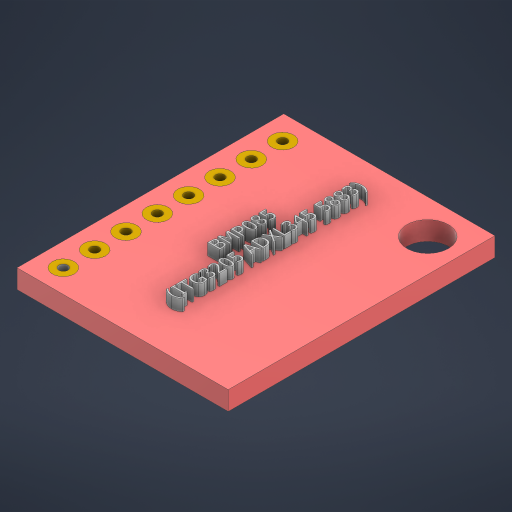
# Autodesk Inventor part: IMU Module
Saved by Autodesk Inventor 2023 (Build 270158000, 158)
## iProperties
Created: 2023-10-20
Part Number: IMU Module
Material: Generic
Document SubType Name: Modeling
Designer: nick_
Density: 1 g/cm^3
Appearance: Default
Author: nick_
Autodesk Inventor part; units mm, degrees
ref_plane "YZ Plane" through (0, 0, 0) normal (1, 0, 0) x (0, 1, 0)
ref_plane "XZ Plane" through (0, 0, 0) normal (0, 1, 0) x (-1, 0, 0)
ref_plane "XY Plane" through (0, 0, 0) normal (0, 0, 1) x (1, 0, 0)
sketch "Sketch1" plane through (0, 0, 0) normal (0, 1, 0) x (-1, 0, 0)
  line L0 (-8.56, 10.81) -> (8.56, 10.81)
  line L1 (8.56, 10.81) -> (8.56, -10.81)
  line L2 (8.56, -10.81) -> (-8.56, -10.81)
  line L3 (-8.56, -10.81) -> (-8.56, 10.81)
  line L4 (-8.56, 10.81) -> (8.56, -10.81) construction
  line L5 (8.56, 10.81) -> (-8.56, -10.81) construction
  point P0 (0, 0)
  dimension "d0" = 17.12
  dimension "d1" = 21.62
  constraints: 12 end point, 2 midpoint, 2 parallel, 1 horizontal, 1 perpendicular
  measures "d0" distance of L1.end L2.end
  measures "d1" distance of L0.end L1.end
extrude "Extrusion1" add sketch "Sketch1" along normal blind 1.53
sketch "Sketch2" plane through (0, 1.53, 0) normal (0, 1, 0) x (1, 0, 0)
  line L0 (8.56, -10.81) -> (8.56, 10.81) projected
  line L1 (8.56, 10.81) -> (-8.56, 10.81) projected
  point P0 (0, 0)
  point P1 (5.895, 8.025)
  dimension "d4" = 2.665
  dimension "d5" = 2.785
  measures "d4" distance from line of L0 point (5.895, 8.025)
  measures "d5" distance from line of L1 point (5.895, 8.025)
hole "Hole1" at (5.895, 1.53, -8.025) direction (0, -1, 0) diameter 3.37 end through all
sketch "Sketch3" plane through (0, 1.53, 0) normal (0, 1, 0) x (1, 0, 0)
  line L0 (-8.56, -10.81) -> (8.56, -10.81) projected
  line L1 (-8.56, 10.81) -> (-8.56, -10.81) projected
  point P0 (0, 0)
  point P1 (-6.685, -8.935)
  dimension "d13" = 1.875
  dimension "d14" = 1.875
  measures "d13" distance from line of L0 point (-6.685, -8.935)
  measures "d14" distance from line of L1 point (-6.685, -8.935)
hole "Hole2" at (-6.685, 1.53, 8.935) direction (0, -1, 0) diameter 0.73 end through all
sketch "Sketch5" plane through (0, 1.53, 0) normal (0, 1, 0) x (1, 0, 0)
  circle A0 centre (-6.685, -8.935) radius 0.365 projected
  circle A1 centre (5.895, 8.025) radius 1.685 construction
  line L0 (8.56, 10.81) -> (-8.56, 10.81) construction
  line L1 (-8.56, 10.81) -> (-8.56, -10.81) construction
  line L2 (-8.56, -10.81) -> (8.56, -10.81) construction
  line L3 (8.56, -10.81) -> (8.56, 10.81) construction
  circle A2 centre (-6.685, -8.935) radius 0.365 construction
  circle A3 centre (-6.685, -8.935) radius 0.885
  point P0 (0, 0)
  dimension "d22" = 1.77
  constraints: 2 coincident, 1 centre point
  measures "d22" diameter of A3
extrude "Extrusion2" add sketch "Sketch5" along normal blind 0.001
pattern_linear "Rectangular Pattern1" count 8 spacing 2.54 along (0, 0, -1) of "Extrusion2", "Hole2"
sketch "Sketch6" plane through (0, 1.53, 0) normal (0, 1, 0) x (1, 0, 0)
  line L0 (-1.7084, -23.5263) -> (-1.7084, 24.1475) construction
  line L1 (-1.7084, 24.1475) -> (7.2695, 24.1475) construction
  line L2 (7.2695, 24.1475) -> (7.2695, -23.5263) construction
  line L3 (7.2695, -23.5263) -> (-1.7084, -23.5263) construction
  spline S0 degree 2 poles (-0.9929, -1.5646) (-0.9183, -1.5646) (-0.804, -1.6213) (-0.7668, -1.6683) knots 0 0 0 1 2 2 2
  spline S1 degree 2 poles (-0.7668, -1.6683) (-0.723, -1.725) (-0.6857, -1.8539) (-0.6857, -1.956) knots 0 0 0 1 2 2 2
  line L4 (-0.6857, -1.956) -> (-0.6857, -2.2429)
  line L5 (-0.6857, -2.2429) -> (-1.6857, -2.2429)
  line L6 (-1.6857, -2.2429) -> (-1.6857, -1.9779)
  spline S2 degree 2 poles (-1.6857, -1.9779) (-1.6857, -1.8709) (-1.672, -1.7639) (-1.6452, -1.7153) knots 0 0 0 1 2 2 2
  spline S3 degree 2 poles (-1.6452, -1.7153) (-1.6169, -1.661) (-1.5237, -1.6116) (-1.4605, -1.6116) knots 0 0 0 1 2 2 2
  spline S4 degree 2 poles (-1.4605, -1.6116) (-1.3899, -1.6116) (-1.2781, -1.6861) (-1.2465, -1.7518) knots 0 0 0 1 2 2 2
  line L7 (-1.2465, -1.7518) -> (-1.2417, -1.7518)
  spline S5 degree 2 poles (-1.2417, -1.7518) (-1.2173, -1.6626) (-1.0885, -1.5646) (-0.9929, -1.5646) knots 0 0 0 1 2 2 2
  spline S6 degree 2 poles (-0.9872, -1.7032) (-1.0439, -1.7032) (-1.1169, -1.7356) (-1.1428, -1.7842) knots 0 0 0 1 2 2 2
  spline S7 degree 2 poles (-1.1428, -1.7842) (-1.159, -1.8158) (-1.1687, -1.8903) (-1.1687, -1.9592) knots 0 0 0 1 2 2 2
  line L8 (-1.1687, -1.9592) -> (-1.1687, -2.11)
  line L9 (-1.1687, -2.11) -> (-0.7992, -2.11)
  line L10 (-0.7992, -2.11) -> (-0.7992, -2.0022)
  spline S8 degree 2 poles (-0.7992, -2.0022) (-0.7992, -1.9147) (-0.8154, -1.8142) (-0.8413, -1.7753) knots 0 0 0 1 2 2 2
  spline S9 degree 2 poles (-0.8413, -1.7753) (-0.8681, -1.738) (-0.9345, -1.7032) (-0.9872, -1.7032) knots 0 0 0 1 2 2 2
  spline S10 degree 2 poles (-1.4418, -1.7502) (-1.4775, -1.7502) (-1.531, -1.7745) (-1.5464, -1.8012) knots 0 0 0 1 2 2 2
  spline S11 degree 2 poles (-1.5464, -1.8012) (-1.5642, -1.8336) (-1.5723, -1.9122) (-1.5723, -1.9827) knots 0 0 0 1 2 2 2
  line L11 (-1.5723, -1.9827) -> (-1.5723, -2.11)
  line L12 (-1.5723, -2.11) -> (-1.2797, -2.11)
  line L13 (-1.2797, -2.11) -> (-1.2797, -1.9592)
  spline S12 degree 2 poles (-1.2797, -1.9592) (-1.2797, -1.8968) (-1.2927, -1.8377) (-1.313, -1.8061) knots 0 0 0 1 2 2 2
  spline S13 degree 2 poles (-1.313, -1.8061) (-1.3324, -1.7753) (-1.3948, -1.7502) (-1.4418, -1.7502) knots 0 0 0 1 2 2 2
  line L14 (-0.6857, -0.5751) -> (-0.6857, -0.708)
  line L15 (-0.6857, -0.708) -> (-1.5472, -0.708)
  line L16 (-1.5472, -0.708) -> (-0.9613, -0.969)
  line L17 (-0.9613, -0.969) -> (-0.9613, -1.05)
  line L18 (-0.9613, -1.05) -> (-1.5472, -1.3085)
  line L19 (-1.5472, -1.3085) -> (-0.6857, -1.3085)
  line L20 (-0.6857, -1.3085) -> (-0.6857, -1.4325)
  line L21 (-0.6857, -1.4325) -> (-1.6857, -1.4325)
  line L22 (-1.6857, -1.4325) -> (-1.6857, -1.251)
  line L23 (-1.6857, -1.251) -> (-1.129, -1.0014)
  line L24 (-1.129, -1.0014) -> (-1.6857, -0.7599)
  line L25 (-1.6857, -0.7599) -> (-1.6857, -0.5751)
  line L26 (-1.6857, -0.5751) -> (-0.6857, -0.5751)
  spline S14 degree 2 poles (-1.3843, 0.2596) (-1.3194, 0.2596) (-1.2028, 0.2134) (-1.1622, 0.172) knots 0 0 0 1 2 2 2
  spline S15 degree 2 poles (-1.1622, 0.172) (-1.1112, 0.1202) (-1.0585, -0.02) (-1.0585, -0.127) knots 0 0 0 1 2 2 2
  line L27 (-1.0585, -0.127) -> (-1.0585, -0.2396)
  line L28 (-1.0585, -0.2396) -> (-0.6857, -0.2396)
  line L29 (-0.6857, -0.2396) -> (-0.6857, -0.3725)
  line L30 (-0.6857, -0.3725) -> (-1.6857, -0.3725)
  line L31 (-1.6857, -0.3725) -> (-1.6857, -0.1213)
  spline S16 degree 2 poles (-1.6857, -0.1213) (-1.6857, -0.0322) (-1.6566, 0.0926) (-1.6233, 0.1404) knots 0 0 0 1 2 2 2
  spline S17 degree 2 poles (-1.6233, 0.1404) (-1.5852, 0.1964) (-1.4677, 0.2596) (-1.3843, 0.2596) knots 0 0 0 1 2 2 2
  spline S18 degree 2 poles (-1.3802, 0.121) (-1.4321, 0.121) (-1.5083, 0.0853) (-1.5326, 0.0489) knots 0 0 0 1 2 2 2
  spline S19 degree 2 poles (-1.5326, 0.0489) (-1.5536, 0.0173) (-1.5707, -0.067) (-1.5707, -0.1294) knots 0 0 0 1 2 2 2
  line L32 (-1.5707, -0.1294) -> (-1.5707, -0.2396)
  line L33 (-1.5707, -0.2396) -> (-1.172, -0.2396)
  line L34 (-1.172, -0.2396) -> (-1.172, -0.1489)
  spline S20 degree 2 poles (-1.172, -0.1489) (-1.172, -0.0678) (-1.1979, 0.0319) (-1.2319, 0.0643) knots 0 0 0 1 2 2 2
  spline S21 degree 2 poles (-1.2319, 0.0643) (-1.2619, 0.0943) (-1.3324, 0.121) (-1.3802, 0.121) knots 0 0 0 1 2 2 2
  spline S22 degree 2 poles (-1.1857, 0.98) (-0.9167, 0.98) (-0.6647, 0.8236) (-0.6647, 0.6607) knots 0 0 0 1 2 2 2
  spline S23 degree 2 poles (-0.6647, 0.6607) (-0.6647, 0.4954) (-0.9216, 0.3406) (-1.1849, 0.3406) knots 0 0 0 1 2 2 2
  spline S24 degree 2 poles (-1.1849, 0.3406) (-1.4556, 0.3406) (-1.706, 0.497) (-1.706, 0.6607) knots 0 0 0 1 2 2 2
  spline S25 degree 2 poles (-1.706, 0.6607) (-1.706, 0.8252) (-1.4467, 0.98) (-1.1857, 0.98) knots 0 0 0 1 2 2 2
  spline S26 degree 2 poles (-0.881, 0.8082) (-0.9305, 0.8276) (-1.0828, 0.8438) (-1.1857, 0.8438) knots 0 0 0 1 2 2 2
  spline S27 degree 2 poles (-1.1857, 0.8438) (-1.2887, 0.8438) (-1.4402, 0.8276) (-1.4912, 0.8074) knots 0 0 0 1 2 2 2
  spline S28 degree 2 poles (-1.4912, 0.8074) (-1.5423, 0.7871) (-1.595, 0.7166) (-1.595, 0.6607) knots 0 0 0 1 2 2 2
  spline S29 degree 2 poles (-1.595, 0.6607) (-1.595, 0.6048) (-1.5423, 0.5327) (-1.4896, 0.5116) knots 0 0 0 1 2 2 2
  spline S30 degree 2 poles (-1.4896, 0.5116) (-1.4386, 0.4913) (-1.283, 0.4767) (-1.1849, 0.4767) knots 0 0 0 1 2 2 2
  spline S31 degree 2 poles (-1.1849, 0.4767) (-1.0796, 0.4767) (-0.9386, 0.4897) (-0.8835, 0.5108) knots 0 0 0 1 2 2 2
  spline S32 degree 2 poles (-0.8835, 0.5108) (-0.8316, 0.5302) (-0.7757, 0.6024) (-0.7757, 0.6607) knots 0 0 0 1 2 2 2
  spline S33 degree 2 poles (-0.7757, 0.6607) (-0.7757, 0.7158) (-0.8284, 0.7879) (-0.881, 0.8082) knots 0 0 0 1 2 2 2
  spline S34 degree 2 poles (-0.663, 1.4103) (-0.663, 1.3357) (-0.7076, 1.2134) (-0.7489, 1.1704) knots 0 0 0 1 2 2 2
  spline S35 degree 2 poles (-0.7489, 1.1704) (-0.7895, 1.1283) (-0.8997, 1.0845) (-0.9621, 1.0845) knots 0 0 0 1 2 2 2
  spline S36 degree 2 poles (-0.9621, 1.0845) (-1.0431, 1.0845) (-1.1793, 1.1712) (-1.2198, 1.2539) knots 0 0 0 1 2 2 2
  line L35 (-1.2198, 1.2539) -> (-1.2238, 1.2539)
  spline S37 degree 2 poles (-1.2238, 1.2539) (-1.2668, 1.1802) (-1.3689, 1.1088) (-1.4451, 1.1088) knots 0 0 0 1 2 2 2
  spline S38 degree 2 poles (-1.4451, 1.1088) (-1.5577, 1.1088) (-1.7084, 1.279) (-1.7084, 1.4103) knots 0 0 0 1 2 2 2
  spline S39 degree 2 poles (-1.7084, 1.4103) (-1.7084, 1.5464) (-1.5658, 1.7109) (-1.454, 1.7109) knots 0 0 0 1 2 2 2
  spline S40 degree 2 poles (-1.454, 1.7109) (-1.3867, 1.7109) (-1.2554, 1.6323) (-1.2181, 1.5586) knots 0 0 0 1 2 2 2
  line L36 (-1.2181, 1.5586) -> (-1.2141, 1.5586)
  spline S41 degree 2 poles (-1.2141, 1.5586) (-1.1736, 1.6461) (-1.0569, 1.7361) (-0.9645, 1.7361) knots 0 0 0 1 2 2 2
  spline S42 degree 2 poles (-0.9645, 1.7361) (-0.8365, 1.7361) (-0.663, 1.5497) (-0.663, 1.4103) knots 0 0 0 1 2 2 2
  spline S43 degree 2 poles (-0.9515, 1.5983) (-1.0131, 1.5983) (-1.0861, 1.5497) (-1.1233, 1.4808) knots 0 0 0 1 2 2 2
  spline S44 degree 2 poles (-1.1233, 1.4808) (-1.1363, 1.4581) (-1.1663, 1.3819) (-1.1857, 1.3341) knots 0 0 0 1 2 2 2
  spline S45 degree 2 poles (-1.1857, 1.3341) (-1.1493, 1.279) (-1.0407, 1.2199) (-0.9718, 1.2199) knots 0 0 0 1 2 2 2
  spline S46 degree 2 poles (-0.9718, 1.2199) (-0.881, 1.2199) (-0.7627, 1.3293) (-0.7627, 1.4119) knots 0 0 0 1 2 2 2
  spline S47 degree 2 poles (-0.7627, 1.4119) (-0.7627, 1.4962) (-0.864, 1.5983) (-0.9515, 1.5983) knots 0 0 0 1 2 2 2
  spline S48 degree 2 poles (-1.4523, 1.5797) (-1.5196, 1.5797) (-1.6096, 1.4897) (-1.6096, 1.4095) knots 0 0 0 1 2 2 2
  spline S49 degree 2 poles (-1.6096, 1.4095) (-1.6096, 1.3366) (-1.5293, 1.2434) (-1.4605, 1.2434) knots 0 0 0 1 2 2 2
  spline S50 degree 2 poles (-1.4605, 1.2434) (-1.411, 1.2434) (-1.3421, 1.2912) (-1.3146, 1.339) knots 0 0 0 1 2 2 2
  spline S51 degree 2 poles (-1.3146, 1.339) (-1.3032, 1.3592) (-1.2635, 1.4451) (-1.2522, 1.48) knots 0 0 0 1 2 2 2
  spline S52 degree 2 poles (-1.2522, 1.48) (-1.2968, 1.5383) (-1.3916, 1.5797) (-1.4523, 1.5797) knots 0 0 0 1 2 2 2
  spline S53 degree 2 poles (-1.0034, 2.4646) (-0.9313, 2.4646) (-0.8081, 2.4184) (-0.7627, 2.3763) knots 0 0 0 1 2 2 2
  spline S54 degree 2 poles (-0.7627, 2.3763) (-0.7173, 2.3341) (-0.6647, 2.2085) (-0.6647, 2.1307) knots 0 0 0 1 2 2 2
  spline S55 degree 2 poles (-0.6647, 2.1307) (-0.6647, 2.0594) (-0.6963, 1.92) (-0.7214, 1.869) knots 0 0 0 1 2 2 2
  line L37 (-0.7214, 1.869) -> (-0.8632, 1.869)
  line L38 (-0.8632, 1.869) -> (-0.8632, 1.8787)
  spline S56 degree 2 poles (-0.8632, 1.8787) (-0.8519, 1.8941) (-0.8227, 1.9516) (-0.8097, 1.9865) knots 0 0 0 1 2 2 2
  spline S57 degree 2 poles (-0.8097, 1.9865) (-0.7959, 2.0262) (-0.7805, 2.0918) (-0.7805, 2.1332) knots 0 0 0 1 2 2 2
  spline S58 degree 2 poles (-0.7805, 2.1332) (-0.7805, 2.1737) (-0.8097, 2.2498) (-0.8413, 2.2774) knots 0 0 0 1 2 2 2
  spline S59 degree 2 poles (-0.8413, 2.2774) (-0.8713, 2.3025) (-0.9507, 2.3285) (-1.0042, 2.3285) knots 0 0 0 1 2 2 2
  spline S60 degree 2 poles (-1.0042, 2.3285) (-1.0577, 2.3285) (-1.1258, 2.2993) (-1.1485, 2.2717) knots 0 0 0 1 2 2 2
  spline S61 degree 2 poles (-1.1485, 2.2717) (-1.1736, 2.2434) (-1.1946, 2.1591) (-1.1946, 2.108) knots 0 0 0 1 2 2 2
  spline S62 degree 2 poles (-1.1946, 2.108) (-1.1946, 2.0529) (-1.1776, 1.9435) (-1.1703, 1.9103) knots 0 0 0 1 2 2 2
  line L39 (-1.1703, 1.9103) -> (-1.6857, 1.9103)
  line L40 (-1.6857, 1.9103) -> (-1.6857, 2.4589)
  line L41 (-1.6857, 2.4589) -> (-1.5682, 2.4589)
  line L42 (-1.5682, 2.4589) -> (-1.5682, 2.0391)
  line L43 (-1.5682, 2.0391) -> (-1.3016, 2.0391)
  spline S63 degree 2 poles (-1.3016, 2.0391) (-1.3049, 2.0635) (-1.3073, 2.1105) (-1.3073, 2.1299) knots 0 0 0 1 2 2 2
  spline S64 degree 2 poles (-1.3073, 2.1299) (-1.3073, 2.2069) (-1.2822, 2.3131) (-1.2449, 2.3617) knots 0 0 0 1 2 2 2
  spline S65 degree 2 poles (-1.2449, 2.3617) (-1.2076, 2.4111) (-1.0942, 2.4646) (-1.0034, 2.4646) knots 0 0 0 1 2 2 2
  line L44 (1.2371, -7.0334) -> (1.2371, -7.1874)
  spline S66 degree 2 poles (1.2371, -7.1874) (1.0985, -7.304) (0.7881, -7.4378) (0.5766, -7.4378) knots 0 0 0 1 2 2 2
  spline S67 degree 2 poles (0.5766, -7.4378) (0.37, -7.4378) (0.0547, -7.3057) (-0.0838, -7.1874) knots 0 0 0 1 2 2 2
  line L45 (-0.0838, -7.1874) -> (-0.0838, -7.0334)
  line L46 (-0.0838, -7.0334) -> (-0.0773, -7.0334)
  spline S68 degree 2 poles (-0.0773, -7.0334) (-0.0279, -7.0877) (0.1001, -7.1865) (0.1852, -7.2287) knots 0 0 0 1 2 2 2
  spline S69 degree 2 poles (0.1852, -7.2287) (0.2679, -7.2692) (0.4664, -7.3194) (0.5766, -7.3194) knots 0 0 0 1 2 2 2
  spline S70 degree 2 poles (0.5766, -7.3194) (0.6917, -7.3194) (0.8821, -7.2708) (0.968, -7.2287) knots 0 0 0 1 2 2 2
  spline S71 degree 2 poles (0.968, -7.2287) (1.0507, -7.1882) (1.1844, -7.0852) (1.2306, -7.0334) knots 0 0 0 1 2 2 2
  line L47 (1.2306, -7.0334) -> (1.2371, -7.0334)
  line L48 (0.9607, -6.5334) -> (0.9607, -6.9207)
  line L49 (0.9607, -6.9207) -> (0.8586, -6.9207)
  line L50 (0.8586, -6.9207) -> (0.8586, -6.7935)
  line L51 (0.8586, -6.7935) -> (0.0628, -6.7935)
  line L52 (0.0628, -6.7935) -> (0.0628, -6.9207)
  line L53 (0.0628, -6.9207) -> (-0.0393, -6.9207)
  line L54 (-0.0393, -6.9207) -> (-0.0393, -6.5334)
  line L55 (-0.0393, -6.5334) -> (0.0628, -6.5334)
  line L56 (0.0628, -6.5334) -> (0.0628, -6.6606)
  line L57 (0.0628, -6.6606) -> (0.8586, -6.6606)
  line L58 (0.8586, -6.6606) -> (0.8586, -6.5334)
  line L59 (0.8586, -6.5334) -> (0.9607, -6.5334)
  line L60 (0.9607, -6.1355) -> (0.0791, -6.1355)
  line L61 (0.0791, -6.1355) -> (0.0791, -6.471)
  line L62 (0.0791, -6.471) -> (-0.0393, -6.471)
  line L63 (-0.0393, -6.471) -> (-0.0393, -5.6671)
  line L64 (-0.0393, -5.6671) -> (0.0791, -5.6671)
  line L65 (0.0791, -5.6671) -> (0.0791, -6.0026)
  line L66 (0.0791, -6.0026) -> (0.9607, -6.0026)
  line L67 (0.9607, -6.0026) -> (0.9607, -6.1355)
  spline S72 degree 2 poles (0.9802, -5.1468) (0.9802, -5.253) (0.9154, -5.4288) (0.8497, -5.4921) knots 0 0 0 1 2 2 2
  spline S73 degree 2 poles (0.8497, -5.4921) (0.7833, -5.5553) (0.5872, -5.6225) (0.4599, -5.6225) knots 0 0 0 1 2 2 2
  spline S74 degree 2 poles (0.4599, -5.6225) (0.3392, -5.6225) (0.1479, -5.5545) (0.0799, -5.4912) knots 0 0 0 1 2 2 2
  spline S75 degree 2 poles (0.0799, -5.4912) (0.0142, -5.4305) (-0.0571, -5.2522) (-0.0571, -5.146) knots 0 0 0 1 2 2 2
  spline S76 degree 2 poles (-0.0571, -5.146) (-0.0571, -5.095) (-0.0425, -5.0026) (-0.0295, -4.9604) knots 0 0 0 1 2 2 2
  spline S77 degree 2 poles (-0.0295, -4.9604) (-0.0198, -4.9264) (0.0158, -4.8438) (0.0288, -4.8186) knots 0 0 0 1 2 2 2
  line L68 (0.0288, -4.8186) -> (0.1893, -4.8186)
  line L69 (0.1893, -4.8186) -> (0.1893, -4.83)
  spline S78 degree 2 poles (0.1893, -4.83) (0.1674, -4.8551) (0.1277, -4.9078) (0.105, -4.9564) knots 0 0 0 1 2 2 2
  spline S79 degree 2 poles (0.105, -4.9564) (0.0847, -4.9969) (0.058, -5.1015) (0.058, -5.1614) knots 0 0 0 1 2 2 2
  spline S80 degree 2 poles (0.058, -5.1614) (0.058, -5.3057) (0.2752, -5.4839) (0.4559, -5.4839) knots 0 0 0 1 2 2 2
  spline S81 degree 2 poles (0.4559, -5.4839) (0.5564, -5.4839) (0.7071, -5.4369) (0.759, -5.3924) knots 0 0 0 1 2 2 2
  spline S82 degree 2 poles (0.759, -5.3924) (0.8108, -5.3494) (0.8651, -5.2279) (0.8651, -5.1517) knots 0 0 0 1 2 2 2
  spline S83 degree 2 poles (0.8651, -5.1517) (0.8651, -5.0958) (0.8489, -4.9839) (0.8327, -4.9459) knots 0 0 0 1 2 2 2
  line L70 (0.8327, -4.9459) -> (0.5742, -4.9459)
  line L71 (0.5742, -4.9459) -> (0.5742, -5.1776)
  line L72 (0.5742, -5.1776) -> (0.4575, -5.1776)
  line L73 (0.4575, -5.1776) -> (0.4575, -4.8146)
  line L74 (0.4575, -4.8146) -> (0.8943, -4.8146)
  spline S84 degree 2 poles (0.8943, -4.8146) (0.9056, -4.8397) (0.9405, -4.9256) (0.951, -4.9621) knots 0 0 0 1 2 2 2
  spline S85 degree 2 poles (0.951, -4.9621) (0.9656, -5.0115) (0.9802, -5.0909) (0.9802, -5.1468) knots 0 0 0 1 2 2 2
  spline S86 degree 2 poles (0.0556, -4.4062) (0.0556, -4.4426) (0.0734, -4.5147) (0.0872, -4.5496) knots 0 0 0 1 2 2 2
  spline S87 degree 2 poles (0.0872, -4.5496) (0.1009, -4.582) (0.1301, -4.6298) (0.1431, -4.6485) knots 0 0 0 1 2 2 2
  line L75 (0.1431, -4.6485) -> (0.1431, -4.6566)
  line L76 (0.1431, -4.6566) -> (0.0013, -4.6566)
  spline S88 degree 2 poles (0.0013, -4.6566) (-0.0222, -4.6128) (-0.0603, -4.4629) (-0.0603, -4.3956) knots 0 0 0 1 2 2 2
  spline S89 degree 2 poles (-0.0603, -4.3956) (-0.0603, -4.3275) (-0.0328, -4.2262) (-0.0036, -4.1849) knots 0 0 0 1 2 2 2
  spline S90 degree 2 poles (-0.0036, -4.1849) (0.028, -4.1412) (0.1196, -4.0958) (0.1812, -4.0958) knots 0 0 0 1 2 2 2
  spline S91 degree 2 poles (0.1812, -4.0958) (0.2638, -4.0958) (0.3886, -4.2044) (0.4048, -4.2805) knots 0 0 0 1 2 2 2
  line L77 (0.4048, -4.2805) -> (0.4145, -4.2805)
  spline S92 degree 2 poles (0.4145, -4.2805) (0.421, -4.2489) (0.4502, -4.1768) (0.4794, -4.146) knots 0 0 0 1 2 2 2
  spline S93 degree 2 poles (0.4794, -4.146) (0.5077, -4.1152) (0.5985, -4.0763) (0.6641, -4.0763) knots 0 0 0 1 2 2 2
  spline S94 degree 2 poles (0.6641, -4.0763) (0.7314, -4.0763) (0.8457, -4.1225) (0.8894, -4.1647) knots 0 0 0 1 2 2 2
  spline S95 degree 2 poles (0.8894, -4.1647) (0.9348, -4.2084) (0.9818, -4.3324) (0.9818, -4.411) knots 0 0 0 1 2 2 2
  spline S96 degree 2 poles (0.9818, -4.411) (0.9818, -4.4864) (0.9453, -4.6339) (0.9202, -4.6841) knots 0 0 0 1 2 2 2
  line L78 (0.9202, -4.6841) -> (0.7784, -4.6841)
  line L79 (0.7784, -4.6841) -> (0.7784, -4.6744)
  spline S97 degree 2 poles (0.7784, -4.6744) (0.8092, -4.6322) (0.8659, -4.4896) (0.8659, -4.4191) knots 0 0 0 1 2 2 2
  spline S98 degree 2 poles (0.8659, -4.4191) (0.8659, -4.3778) (0.84, -4.2951) (0.81, -4.2676) knots 0 0 0 1 2 2 2
  spline S99 degree 2 poles (0.81, -4.2676) (0.78, -4.2408) (0.7087, -4.2125) (0.6544, -4.2125) knots 0 0 0 1 2 2 2
  spline S100 degree 2 poles (0.6544, -4.2125) (0.6001, -4.2125) (0.5296, -4.2441) (0.5094, -4.2724) knots 0 0 0 1 2 2 2
  spline S101 degree 2 poles (0.5094, -4.2724) (0.4891, -4.3008) (0.4737, -4.3778) (0.4737, -4.4232) knots 0 0 0 1 2 2 2
  line L80 (0.4737, -4.4232) -> (0.4737, -4.4799)
  line L81 (0.4737, -4.4799) -> (0.3627, -4.4799)
  line L82 (0.3627, -4.4799) -> (0.3627, -4.4353)
  spline S102 degree 2 poles (0.3627, -4.4353) (0.3627, -4.3454) (0.2768, -4.2319) (0.1949, -4.2319) knots 0 0 0 1 2 2 2
  spline S103 degree 2 poles (0.1949, -4.2319) (0.1568, -4.2319) (0.1026, -4.2611) (0.0863, -4.2846) knots 0 0 0 1 2 2 2
  spline S104 degree 2 poles (0.0863, -4.2846) (0.0693, -4.3097) (0.0556, -4.3713) (0.0556, -4.4062) knots 0 0 0 1 2 2 2
  line L83 (0.9607, -3.3089) -> (0.9607, -3.9256)
  line L84 (0.9607, -3.9256) -> (0.8189, -3.9256)
  spline S105 degree 2 poles (0.8189, -3.9256) (0.7565, -3.8592) (0.6406, -3.7408) (0.5782, -3.6841) knots 0 0 0 1 2 2 2
  spline S106 degree 2 poles (0.5782, -3.6841) (0.4526, -3.5698) (0.3019, -3.4864) (0.2217, -3.4864) knots 0 0 0 1 2 2 2
  spline S107 degree 2 poles (0.2217, -3.4864) (0.1795, -3.4864) (0.1163, -3.5123) (0.0961, -3.5358) knots 0 0 0 1 2 2 2
  spline S108 degree 2 poles (0.0961, -3.5358) (0.0758, -3.5593) (0.0556, -3.6209) (0.0556, -3.6582) knots 0 0 0 1 2 2 2
  spline S109 degree 2 poles (0.0556, -3.6582) (0.0556, -3.6938) (0.0734, -3.7668) (0.0872, -3.8) knots 0 0 0 1 2 2 2
  spline S110 degree 2 poles (0.0872, -3.8) (0.0985, -3.8284) (0.1309, -3.881) (0.1423, -3.8972) knots 0 0 0 1 2 2 2
  line L85 (0.1423, -3.8972) -> (0.1423, -3.9045)
  line L86 (0.1423, -3.9045) -> (-0.0004, -3.9045)
  spline S111 degree 2 poles (-0.0004, -3.9045) (-0.0206, -3.8632) (-0.0603, -3.7149) (-0.0603, -3.6485) knots 0 0 0 1 2 2 2
  spline S112 degree 2 poles (-0.0603, -3.6485) (-0.0603, -3.5083) (0.088, -3.3502) (0.2144, -3.3502) knots 0 0 0 1 2 2 2
  spline S113 degree 2 poles (0.2144, -3.3502) (0.2735, -3.3502) (0.3724, -3.3778) (0.4145, -3.4021) knots 0 0 0 1 2 2 2
  spline S114 degree 2 poles (0.4145, -3.4021) (0.4583, -3.4264) (0.5442, -3.4969) (0.5855, -3.5358) knots 0 0 0 1 2 2 2
  spline S115 degree 2 poles (0.5855, -3.5358) (0.6544, -3.599) (0.8019, -3.7538) (0.8449, -3.8) knots 0 0 0 1 2 2 2
  line L87 (0.8449, -3.8) -> (0.8449, -3.3089)
  line L88 (0.8449, -3.3089) -> (0.9607, -3.3089)
  spline S116 degree 2 poles (0.4607, -2.5528) (0.7298, -2.5528) (0.9818, -2.7092) (0.9818, -2.8721) knots 0 0 0 1 2 2 2
  spline S117 degree 2 poles (0.9818, -2.8721) (0.9818, -3.0374) (0.7249, -3.1922) (0.4615, -3.1922) knots 0 0 0 1 2 2 2
  spline S118 degree 2 poles (0.4615, -3.1922) (0.1909, -3.1922) (-0.0595, -3.0358) (-0.0595, -2.8721) knots 0 0 0 1 2 2 2
  spline S119 degree 2 poles (-0.0595, -2.8721) (-0.0595, -2.7076) (0.1998, -2.5528) (0.4607, -2.5528) knots 0 0 0 1 2 2 2
  spline S120 degree 2 poles (0.7654, -2.7246) (0.716, -2.7052) (0.5637, -2.689) (0.4607, -2.689) knots 0 0 0 1 2 2 2
  spline S121 degree 2 poles (0.4607, -2.689) (0.3578, -2.689) (0.2063, -2.7052) (0.1552, -2.7254) knots 0 0 0 1 2 2 2
  spline S122 degree 2 poles (0.1552, -2.7254) (0.1042, -2.7457) (0.0515, -2.8162) (0.0515, -2.8721) knots 0 0 0 1 2 2 2
  spline S123 degree 2 poles (0.0515, -2.8721) (0.0515, -2.928) (0.1042, -3.0002) (0.1568, -3.0212) knots 0 0 0 1 2 2 2
  spline S124 degree 2 poles (0.1568, -3.0212) (0.2079, -3.0415) (0.3635, -3.0561) (0.4615, -3.0561) knots 0 0 0 1 2 2 2
  spline S125 degree 2 poles (0.4615, -3.0561) (0.5669, -3.0561) (0.7079, -3.0431) (0.763, -3.022) knots 0 0 0 1 2 2 2
  spline S126 degree 2 poles (0.763, -3.022) (0.8149, -3.0026) (0.8708, -2.9305) (0.8708, -2.8721) knots 0 0 0 1 2 2 2
  spline S127 degree 2 poles (0.8708, -2.8721) (0.8708, -2.817) (0.8181, -2.7449) (0.7654, -2.7246) knots 0 0 0 1 2 2 2
  spline S128 degree 2 poles (0.6431, -1.8186) (0.7152, -1.8186) (0.8384, -1.8648) (0.8838, -1.907) knots 0 0 0 1 2 2 2
  spline S129 degree 2 poles (0.8838, -1.907) (0.9291, -1.9491) (0.9818, -2.0747) (0.9818, -2.1525) knots 0 0 0 1 2 2 2
  spline S130 degree 2 poles (0.9818, -2.1525) (0.9818, -2.2238) (0.9502, -2.3632) (0.9251, -2.4143) knots 0 0 0 1 2 2 2
  line L89 (0.9251, -2.4143) -> (0.7833, -2.4143)
  line L90 (0.7833, -2.4143) -> (0.7833, -2.4045)
  spline S131 degree 2 poles (0.7833, -2.4045) (0.7946, -2.3891) (0.8238, -2.3316) (0.8368, -2.2968) knots 0 0 0 1 2 2 2
  spline S132 degree 2 poles (0.8368, -2.2968) (0.8505, -2.257) (0.8659, -2.1914) (0.8659, -2.1501) knots 0 0 0 1 2 2 2
  spline S133 degree 2 poles (0.8659, -2.1501) (0.8659, -2.1096) (0.8368, -2.0334) (0.8051, -2.0058) knots 0 0 0 1 2 2 2
  spline S134 degree 2 poles (0.8051, -2.0058) (0.7752, -1.9807) (0.6957, -1.9548) (0.6423, -1.9548) knots 0 0 0 1 2 2 2
  spline S135 degree 2 poles (0.6423, -1.9548) (0.5888, -1.9548) (0.5207, -1.9839) (0.498, -2.0115) knots 0 0 0 1 2 2 2
  spline S136 degree 2 poles (0.498, -2.0115) (0.4729, -2.0399) (0.4518, -2.1241) (0.4518, -2.1752) knots 0 0 0 1 2 2 2
  spline S137 degree 2 poles (0.4518, -2.1752) (0.4518, -2.2303) (0.4688, -2.3397) (0.4761, -2.3729) knots 0 0 0 1 2 2 2
  line L91 (0.4761, -2.3729) -> (-0.0393, -2.3729)
  line L92 (-0.0393, -2.3729) -> (-0.0393, -1.8243)
  line L93 (-0.0393, -1.8243) -> (0.0782, -1.8243)
  line L94 (0.0782, -1.8243) -> (0.0782, -2.2441)
  line L95 (0.0782, -2.2441) -> (0.3449, -2.2441)
  spline S138 degree 2 poles (0.3449, -2.2441) (0.3416, -2.2198) (0.3392, -2.1728) (0.3392, -2.1533) knots 0 0 0 1 2 2 2
  spline S139 degree 2 poles (0.3392, -2.1533) (0.3392, -2.0763) (0.3643, -1.9702) (0.4016, -1.9215) knots 0 0 0 1 2 2 2
  spline S140 degree 2 poles (0.4016, -1.9215) (0.4389, -1.8721) (0.5523, -1.8186) (0.6431, -1.8186) knots 0 0 0 1 2 2 2
  line L96 (0.9607, -1.3243) -> (-0.0393, -0.9872)
  line L97 (-0.0393, -0.9872) -> (-0.0393, -0.8235)
  line L98 (-0.0393, -0.8235) -> (0.9607, -0.4864)
  line L99 (0.9607, -0.4864) -> (0.9607, -0.6266)
  line L100 (0.9607, -0.6266) -> (0.6812, -0.7173)
  line L101 (0.6812, -0.7173) -> (0.6812, -1.099)
  line L102 (0.6812, -1.099) -> (0.9607, -1.1898)
  line L103 (0.9607, -1.1898) -> (0.9607, -1.3243)
  line L104 (0.5677, -0.7538) -> (0.0969, -0.9086)
  line L105 (0.0969, -0.9086) -> (0.5677, -1.0626)
  line L106 (0.5677, -1.0626) -> (0.5677, -0.7538)
  spline S141 degree 2 poles (0.4615, 0.3969) (0.5985, 0.3969) (0.8189, 0.2859) (0.8805, 0.1927) knots 0 0 0 1 2 2 2
  spline S142 degree 2 poles (0.8805, 0.1927) (0.9283, 0.1165) (0.9607, -0.0399) (0.9607, -0.1614) knots 0 0 0 1 2 2 2
  line L107 (0.9607, -0.1614) -> (0.9607, -0.3916)
  line L108 (0.9607, -0.3916) -> (-0.0393, -0.3916)
  line L109 (-0.0393, -0.3916) -> (-0.0393, -0.1639)
  spline S143 degree 2 poles (-0.0393, -0.1639) (-0.0393, -0.0228) (0.0029, 0.1376) (0.0402, 0.1943) knots 0 0 0 1 2 2 2
  spline S144 degree 2 poles (0.0402, 0.1943) (0.1042, 0.2908) (0.3157, 0.3969) (0.4615, 0.3969) knots 0 0 0 1 2 2 2
  spline S145 degree 2 poles (0.4599, 0.2584) (0.3449, 0.2584) (0.182, 0.1822) (0.1358, 0.1068) knots 0 0 0 1 2 2 2
  spline S146 degree 2 poles (0.1358, 0.1068) (0.1042, 0.0533) (0.0758, -0.0674) (0.0758, -0.1574) knots 0 0 0 1 2 2 2
  line L110 (0.0758, -0.1574) -> (0.0758, -0.2587)
  line L111 (0.0758, -0.2587) -> (0.8457, -0.2587)
  line L112 (0.8457, -0.2587) -> (0.8457, -0.1574)
  spline S147 degree 2 poles (0.8457, -0.1574) (0.8457, -0.069) (0.8173, 0.0647) (0.7792, 0.119) knots 0 0 0 1 2 2 2
  spline S148 degree 2 poles (0.7792, 0.119) (0.7322, 0.1887) (0.5766, 0.2584) (0.4599, 0.2584) knots 0 0 0 1 2 2 2
  line L113 (0.9607, 1.2324) -> (0.9607, 1.0801)
  line L114 (0.9607, 1.0801) -> (0.562, 0.837)
  line L115 (0.562, 0.837) -> (0.9607, 0.589)
  line L116 (0.9607, 0.589) -> (0.9607, 0.4455)
  line L117 (0.9607, 0.4455) -> (0.4599, 0.764)
  line L118 (0.4599, 0.764) -> (-0.0393, 0.4553)
  line L119 (-0.0393, 0.4553) -> (-0.0393, 0.6076)
  line L120 (-0.0393, 0.6076) -> (0.3521, 0.8459)
  line L121 (0.3521, 0.8459) -> (-0.0393, 1.089)
  line L122 (-0.0393, 1.089) -> (-0.0393, 1.2324)
  line L123 (-0.0393, 1.2324) -> (0.4534, 0.9196)
  line L124 (0.4534, 0.9196) -> (0.9607, 1.2324)
  line L125 (0.9607, 1.9188) -> (0.9607, 1.3394)
  line L126 (0.9607, 1.3394) -> (-0.0393, 1.3394)
  line L127 (-0.0393, 1.3394) -> (-0.0393, 1.4723)
  line L128 (-0.0393, 1.4723) -> (0.8424, 1.4723)
  line L129 (0.8424, 1.4723) -> (0.8424, 1.9188)
  line L130 (0.8424, 1.9188) -> (0.9607, 1.9188)
  spline S149 degree 2 poles (0.0556, 2.2648) (0.0556, 2.2284) (0.0734, 2.1562) (0.0872, 2.1214) knots 0 0 0 1 2 2 2
  spline S150 degree 2 poles (0.0872, 2.1214) (0.1009, 2.089) (0.1301, 2.0412) (0.1431, 2.0225) knots 0 0 0 1 2 2 2
  line L131 (0.1431, 2.0225) -> (0.1431, 2.0144)
  line L132 (0.1431, 2.0144) -> (0.0013, 2.0144)
  spline S151 degree 2 poles (0.0013, 2.0144) (-0.0222, 2.0582) (-0.0603, 2.2081) (-0.0603, 2.2754) knots 0 0 0 1 2 2 2
  spline S152 degree 2 poles (-0.0603, 2.2754) (-0.0603, 2.3434) (-0.0328, 2.4447) (-0.0036, 2.4861) knots 0 0 0 1 2 2 2
  spline S153 degree 2 poles (-0.0036, 2.4861) (0.028, 2.5298) (0.1196, 2.5752) (0.1812, 2.5752) knots 0 0 0 1 2 2 2
  spline S154 degree 2 poles (0.1812, 2.5752) (0.2638, 2.5752) (0.3886, 2.4666) (0.4048, 2.3904) knots 0 0 0 1 2 2 2
  line L133 (0.4048, 2.3904) -> (0.4145, 2.3904)
  spline S155 degree 2 poles (0.4145, 2.3904) (0.421, 2.422) (0.4502, 2.4942) (0.4794, 2.525) knots 0 0 0 1 2 2 2
  spline S156 degree 2 poles (0.4794, 2.525) (0.5077, 2.5558) (0.5985, 2.5947) (0.6641, 2.5947) knots 0 0 0 1 2 2 2
  spline S157 degree 2 poles (0.6641, 2.5947) (0.7314, 2.5947) (0.8457, 2.5485) (0.8894, 2.5063) knots 0 0 0 1 2 2 2
  spline S158 degree 2 poles (0.8894, 2.5063) (0.9348, 2.4626) (0.9818, 2.3386) (0.9818, 2.26) knots 0 0 0 1 2 2 2
  spline S159 degree 2 poles (0.9818, 2.26) (0.9818, 2.1846) (0.9453, 2.0371) (0.9202, 1.9869) knots 0 0 0 1 2 2 2
  line L134 (0.9202, 1.9869) -> (0.7784, 1.9869)
  line L135 (0.7784, 1.9869) -> (0.7784, 1.9966)
  spline S160 degree 2 poles (0.7784, 1.9966) (0.8092, 2.0387) (0.8659, 2.1814) (0.8659, 2.2519) knots 0 0 0 1 2 2 2
  spline S161 degree 2 poles (0.8659, 2.2519) (0.8659, 2.2932) (0.84, 2.3759) (0.81, 2.4034) knots 0 0 0 1 2 2 2
  spline S162 degree 2 poles (0.81, 2.4034) (0.78, 2.4302) (0.7087, 2.4585) (0.6544, 2.4585) knots 0 0 0 1 2 2 2
  spline S163 degree 2 poles (0.6544, 2.4585) (0.6001, 2.4585) (0.5296, 2.4269) (0.5094, 2.3985) knots 0 0 0 1 2 2 2
  spline S164 degree 2 poles (0.5094, 2.3985) (0.4891, 2.3702) (0.4737, 2.2932) (0.4737, 2.2478) knots 0 0 0 1 2 2 2
  line L136 (0.4737, 2.2478) -> (0.4737, 2.1911)
  line L137 (0.4737, 2.1911) -> (0.3627, 2.1911)
  line L138 (0.3627, 2.1911) -> (0.3627, 2.2357)
  spline S165 degree 2 poles (0.3627, 2.2357) (0.3627, 2.3256) (0.2768, 2.4391) (0.1949, 2.4391) knots 0 0 0 1 2 2 2
  spline S166 degree 2 poles (0.1949, 2.4391) (0.1568, 2.4391) (0.1026, 2.4099) (0.0863, 2.3864) knots 0 0 0 1 2 2 2
  spline S167 degree 2 poles (0.0863, 2.3864) (0.0693, 2.3613) (0.0556, 2.2997) (0.0556, 2.2648) knots 0 0 0 1 2 2 2
  line L139 (0.6171, 3.3888) -> (0.6171, 3.2697)
  line L140 (0.6171, 3.2697) -> (0.9607, 3.2697)
  line L141 (0.9607, 3.2697) -> (0.9607, 3.1408)
  line L142 (0.9607, 3.1408) -> (0.6171, 3.1408)
  line L143 (0.6171, 3.1408) -> (0.6171, 2.6992)
  line L144 (0.6171, 2.6992) -> (0.4761, 2.6992)
  line L145 (0.4761, 2.6992) -> (-0.0393, 3.1465)
  line L146 (-0.0393, 3.1465) -> (-0.0393, 3.2697)
  line L147 (-0.0393, 3.2697) -> (0.5094, 3.2697)
  line L148 (0.5094, 3.2697) -> (0.5094, 3.3888)
  line L149 (0.5094, 3.3888) -> (0.6171, 3.3888)
  line L150 (0.5094, 3.1408) -> (0.1188, 3.1408)
  line L151 (0.1188, 3.1408) -> (0.5094, 2.8045)
  line L152 (0.5094, 2.8045) -> (0.5094, 3.1408)
  spline S168 degree 2 poles (0.6431, 4.102) (0.7152, 4.102) (0.8384, 4.0558) (0.8838, 4.0136) knots 0 0 0 1 2 2 2
  spline S169 degree 2 poles (0.8838, 4.0136) (0.9291, 3.9715) (0.9818, 3.8459) (0.9818, 3.7681) knots 0 0 0 1 2 2 2
  spline S170 degree 2 poles (0.9818, 3.7681) (0.9818, 3.6968) (0.9502, 3.5574) (0.9251, 3.5063) knots 0 0 0 1 2 2 2
  line L153 (0.9251, 3.5063) -> (0.7833, 3.5063)
  line L154 (0.7833, 3.5063) -> (0.7833, 3.5161)
  spline S171 degree 2 poles (0.7833, 3.5161) (0.7946, 3.5314) (0.8238, 3.589) (0.8368, 3.6238) knots 0 0 0 1 2 2 2
  spline S172 degree 2 poles (0.8368, 3.6238) (0.8505, 3.6635) (0.8659, 3.7292) (0.8659, 3.7705) knots 0 0 0 1 2 2 2
  spline S173 degree 2 poles (0.8659, 3.7705) (0.8659, 3.811) (0.8368, 3.8872) (0.8051, 3.9148) knots 0 0 0 1 2 2 2
  spline S174 degree 2 poles (0.8051, 3.9148) (0.7752, 3.9399) (0.6957, 3.9658) (0.6423, 3.9658) knots 0 0 0 1 2 2 2
  spline S175 degree 2 poles (0.6423, 3.9658) (0.5888, 3.9658) (0.5207, 3.9366) (0.498, 3.9091) knots 0 0 0 1 2 2 2
  spline S176 degree 2 poles (0.498, 3.9091) (0.4729, 3.8807) (0.4518, 3.7964) (0.4518, 3.7454) knots 0 0 0 1 2 2 2
  spline S177 degree 2 poles (0.4518, 3.7454) (0.4518, 3.6903) (0.4688, 3.5809) (0.4761, 3.5477) knots 0 0 0 1 2 2 2
  line L155 (0.4761, 3.5477) -> (-0.0393, 3.5477)
  line L156 (-0.0393, 3.5477) -> (-0.0393, 4.0963)
  line L157 (-0.0393, 4.0963) -> (0.0782, 4.0963)
  line L158 (0.0782, 4.0963) -> (0.0782, 3.6765)
  line L159 (0.0782, 3.6765) -> (0.3449, 3.6765)
  spline S178 degree 2 poles (0.3449, 3.6765) (0.3416, 3.7008) (0.3392, 3.7478) (0.3392, 3.7673) knots 0 0 0 1 2 2 2
  spline S179 degree 2 poles (0.3392, 3.7673) (0.3392, 3.8443) (0.3643, 3.9504) (0.4016, 3.999) knots 0 0 0 1 2 2 2
  spline S180 degree 2 poles (0.4016, 3.999) (0.4389, 4.0485) (0.5523, 4.102) (0.6431, 4.102) knots 0 0 0 1 2 2 2
  spline S181 degree 2 poles (0.6431, 5.2819) (0.7152, 5.2819) (0.8384, 5.2357) (0.8838, 5.1935) knots 0 0 0 1 2 2 2
  spline S182 degree 2 poles (0.8838, 5.1935) (0.9291, 5.1514) (0.9818, 5.0258) (0.9818, 4.948) knots 0 0 0 1 2 2 2
  spline S183 degree 2 poles (0.9818, 4.948) (0.9818, 4.8767) (0.9502, 4.7373) (0.9251, 4.6862) knots 0 0 0 1 2 2 2
  line L160 (0.9251, 4.6862) -> (0.7833, 4.6862)
  line L161 (0.7833, 4.6862) -> (0.7833, 4.696)
  spline S184 degree 2 poles (0.7833, 4.696) (0.7946, 4.7114) (0.8238, 4.7689) (0.8368, 4.8037) knots 0 0 0 1 2 2 2
  spline S185 degree 2 poles (0.8368, 4.8037) (0.8505, 4.8434) (0.8659, 4.9091) (0.8659, 4.9504) knots 0 0 0 1 2 2 2
  spline S186 degree 2 poles (0.8659, 4.9504) (0.8659, 4.9909) (0.8368, 5.0671) (0.8051, 5.0947) knots 0 0 0 1 2 2 2
  spline S187 degree 2 poles (0.8051, 5.0947) (0.7752, 5.1198) (0.6957, 5.1457) (0.6423, 5.1457) knots 0 0 0 1 2 2 2
  spline S188 degree 2 poles (0.6423, 5.1457) (0.5888, 5.1457) (0.5207, 5.1165) (0.498, 5.089) knots 0 0 0 1 2 2 2
  spline S189 degree 2 poles (0.498, 5.089) (0.4729, 5.0606) (0.4518, 4.9763) (0.4518, 4.9253) knots 0 0 0 1 2 2 2
  spline S190 degree 2 poles (0.4518, 4.9253) (0.4518, 4.8702) (0.4688, 4.7608) (0.4761, 4.7276) knots 0 0 0 1 2 2 2
  line L162 (0.4761, 4.7276) -> (-0.0393, 4.7276)
  line L163 (-0.0393, 4.7276) -> (-0.0393, 5.2762)
  line L164 (-0.0393, 5.2762) -> (0.0782, 5.2762)
  line L165 (0.0782, 5.2762) -> (0.0782, 4.8564)
  line L166 (0.0782, 4.8564) -> (0.3449, 4.8564)
  spline S191 degree 2 poles (0.3449, 4.8564) (0.3416, 4.8807) (0.3392, 4.9277) (0.3392, 4.9472) knots 0 0 0 1 2 2 2
  spline S192 degree 2 poles (0.3392, 4.9472) (0.3392, 5.0242) (0.3643, 5.1303) (0.4016, 5.1789) knots 0 0 0 1 2 2 2
  spline S193 degree 2 poles (0.4016, 5.1789) (0.4389, 5.2284) (0.5523, 5.2819) (0.6431, 5.2819) knots 0 0 0 1 2 2 2
  spline S194 degree 2 poles (0.9834, 5.7284) (0.9834, 5.6538) (0.9389, 5.5314) (0.8975, 5.4885) knots 0 0 0 1 2 2 2
  spline S195 degree 2 poles (0.8975, 5.4885) (0.857, 5.4464) (0.7468, 5.4026) (0.6844, 5.4026) knots 0 0 0 1 2 2 2
  spline S196 degree 2 poles (0.6844, 5.4026) (0.6034, 5.4026) (0.4672, 5.4893) (0.4267, 5.572) knots 0 0 0 1 2 2 2
  line L167 (0.4267, 5.572) -> (0.4227, 5.572)
  spline S197 degree 2 poles (0.4227, 5.572) (0.3797, 5.4982) (0.2776, 5.4269) (0.2014, 5.4269) knots 0 0 0 1 2 2 2
  spline S198 degree 2 poles (0.2014, 5.4269) (0.0888, 5.4269) (-0.062, 5.5971) (-0.062, 5.7284) knots 0 0 0 1 2 2 2
  spline S199 degree 2 poles (-0.062, 5.7284) (-0.062, 5.8645) (0.0807, 6.029) (0.1925, 6.029) knots 0 0 0 1 2 2 2
  spline S200 degree 2 poles (0.1925, 6.029) (0.2598, 6.029) (0.391, 5.9504) (0.4283, 5.8767) knots 0 0 0 1 2 2 2
  line L168 (0.4283, 5.8767) -> (0.4324, 5.8767)
  spline S201 degree 2 poles (0.4324, 5.8767) (0.4729, 5.9642) (0.5896, 6.0541) (0.682, 6.0541) knots 0 0 0 1 2 2 2
  spline S202 degree 2 poles (0.682, 6.0541) (0.81, 6.0541) (0.9834, 5.8678) (0.9834, 5.7284) knots 0 0 0 1 2 2 2
  spline S203 degree 2 poles (0.6949, 5.9164) (0.6333, 5.9164) (0.5604, 5.8678) (0.5231, 5.7989) knots 0 0 0 1 2 2 2
  spline S204 degree 2 poles (0.5231, 5.7989) (0.5102, 5.7762) (0.4802, 5.7) (0.4607, 5.6522) knots 0 0 0 1 2 2 2
  spline S205 degree 2 poles (0.4607, 5.6522) (0.4972, 5.5971) (0.6058, 5.5379) (0.6747, 5.5379) knots 0 0 0 1 2 2 2
  spline S206 degree 2 poles (0.6747, 5.5379) (0.7654, 5.5379) (0.8838, 5.6473) (0.8838, 5.73) knots 0 0 0 1 2 2 2
  spline S207 degree 2 poles (0.8838, 5.73) (0.8838, 5.8143) (0.7825, 5.9164) (0.6949, 5.9164) knots 0 0 0 1 2 2 2
  spline S208 degree 2 poles (0.1941, 5.8977) (0.1269, 5.8977) (0.0369, 5.8078) (0.0369, 5.7276) knots 0 0 0 1 2 2 2
  spline S209 degree 2 poles (0.0369, 5.7276) (0.0369, 5.6546) (0.1171, 5.5614) (0.186, 5.5614) knots 0 0 0 1 2 2 2
  spline S210 degree 2 poles (0.186, 5.5614) (0.2355, 5.5614) (0.3043, 5.6092) (0.3319, 5.6571) knots 0 0 0 1 2 2 2
  spline S211 degree 2 poles (0.3319, 5.6571) (0.3432, 5.6773) (0.3829, 5.7632) (0.3943, 5.7981) knots 0 0 0 1 2 2 2
  spline S212 degree 2 poles (0.3943, 5.7981) (0.3497, 5.8564) (0.2549, 5.8977) (0.1941, 5.8977) knots 0 0 0 1 2 2 2
  spline S213 degree 2 poles (0.9834, 6.4788) (0.9834, 6.4042) (0.9389, 6.2819) (0.8975, 6.2389) knots 0 0 0 1 2 2 2
  spline S214 degree 2 poles (0.8975, 6.2389) (0.857, 6.1968) (0.7468, 6.153) (0.6844, 6.153) knots 0 0 0 1 2 2 2
  spline S215 degree 2 poles (0.6844, 6.153) (0.6034, 6.153) (0.4672, 6.2397) (0.4267, 6.3224) knots 0 0 0 1 2 2 2
  line L169 (0.4267, 6.3224) -> (0.4227, 6.3224)
  spline S216 degree 2 poles (0.4227, 6.3224) (0.3797, 6.2486) (0.2776, 6.1773) (0.2014, 6.1773) knots 0 0 0 1 2 2 2
  spline S217 degree 2 poles (0.2014, 6.1773) (0.0888, 6.1773) (-0.062, 6.3475) (-0.062, 6.4788) knots 0 0 0 1 2 2 2
  spline S218 degree 2 poles (-0.062, 6.4788) (-0.062, 6.6149) (0.0807, 6.7794) (0.1925, 6.7794) knots 0 0 0 1 2 2 2
  spline S219 degree 2 poles (0.1925, 6.7794) (0.2598, 6.7794) (0.391, 6.7008) (0.4283, 6.6271) knots 0 0 0 1 2 2 2
  line L170 (0.4283, 6.6271) -> (0.4324, 6.6271)
  spline S220 degree 2 poles (0.4324, 6.6271) (0.4729, 6.7146) (0.5896, 6.8045) (0.682, 6.8045) knots 0 0 0 1 2 2 2
  spline S221 degree 2 poles (0.682, 6.8045) (0.81, 6.8045) (0.9834, 6.6182) (0.9834, 6.4788) knots 0 0 0 1 2 2 2
  spline S222 degree 2 poles (0.6949, 6.6668) (0.6333, 6.6668) (0.5604, 6.6182) (0.5231, 6.5493) knots 0 0 0 1 2 2 2
  spline S223 degree 2 poles (0.5231, 6.5493) (0.5102, 6.5266) (0.4802, 6.4504) (0.4607, 6.4026) knots 0 0 0 1 2 2 2
  spline S224 degree 2 poles (0.4607, 6.4026) (0.4972, 6.3475) (0.6058, 6.2883) (0.6747, 6.2883) knots 0 0 0 1 2 2 2
  spline S225 degree 2 poles (0.6747, 6.2883) (0.7654, 6.2883) (0.8838, 6.3977) (0.8838, 6.4804) knots 0 0 0 1 2 2 2
  spline S226 degree 2 poles (0.8838, 6.4804) (0.8838, 6.5647) (0.7825, 6.6668) (0.6949, 6.6668) knots 0 0 0 1 2 2 2
  spline S227 degree 2 poles (0.1941, 6.6481) (0.1269, 6.6481) (0.0369, 6.5582) (0.0369, 6.478) knots 0 0 0 1 2 2 2
  spline S228 degree 2 poles (0.0369, 6.478) (0.0369, 6.405) (0.1171, 6.3118) (0.186, 6.3118) knots 0 0 0 1 2 2 2
  spline S229 degree 2 poles (0.186, 6.3118) (0.2355, 6.3118) (0.3043, 6.3597) (0.3319, 6.4075) knots 0 0 0 1 2 2 2
  spline S230 degree 2 poles (0.3319, 6.4075) (0.3432, 6.4277) (0.3829, 6.5136) (0.3943, 6.5485) knots 0 0 0 1 2 2 2
  spline S231 degree 2 poles (0.3943, 6.5485) (0.3497, 6.6068) (0.2549, 6.6481) (0.1941, 6.6481) knots 0 0 0 1 2 2 2
  spline S232 degree 2 poles (0.0556, 7.1968) (0.0556, 7.1603) (0.0734, 7.0882) (0.0872, 7.0533) knots 0 0 0 1 2 2 2
  spline S233 degree 2 poles (0.0872, 7.0533) (0.1009, 7.0209) (0.1301, 6.9731) (0.1431, 6.9545) knots 0 0 0 1 2 2 2
  line L171 (0.1431, 6.9545) -> (0.1431, 6.9464)
  line L172 (0.1431, 6.9464) -> (0.0013, 6.9464)
  spline S234 degree 2 poles (0.0013, 6.9464) (-0.0222, 6.9901) (-0.0603, 7.14) (-0.0603, 7.2073) knots 0 0 0 1 2 2 2
  spline S235 degree 2 poles (-0.0603, 7.2073) (-0.0603, 7.2754) (-0.0328, 7.3767) (-0.0036, 7.418) knots 0 0 0 1 2 2 2
  spline S236 degree 2 poles (-0.0036, 7.418) (0.028, 7.4618) (0.1196, 7.5071) (0.1812, 7.5071) knots 0 0 0 1 2 2 2
  spline S237 degree 2 poles (0.1812, 7.5071) (0.2638, 7.5071) (0.3886, 7.3985) (0.4048, 7.3224) knots 0 0 0 1 2 2 2
  line L173 (0.4048, 7.3224) -> (0.4145, 7.3224)
  spline S238 degree 2 poles (0.4145, 7.3224) (0.421, 7.354) (0.4502, 7.4261) (0.4794, 7.4569) knots 0 0 0 1 2 2 2
  spline S239 degree 2 poles (0.4794, 7.4569) (0.5077, 7.4877) (0.5985, 7.5266) (0.6641, 7.5266) knots 0 0 0 1 2 2 2
  spline S240 degree 2 poles (0.6641, 7.5266) (0.7314, 7.5266) (0.8457, 7.4804) (0.8894, 7.4383) knots 0 0 0 1 2 2 2
  spline S241 degree 2 poles (0.8894, 7.4383) (0.9348, 7.3945) (0.9818, 7.2705) (0.9818, 7.1919) knots 0 0 0 1 2 2 2
  spline S242 degree 2 poles (0.9818, 7.1919) (0.9818, 7.1165) (0.9453, 6.9691) (0.9202, 6.9188) knots 0 0 0 1 2 2 2
  line L174 (0.9202, 6.9188) -> (0.7784, 6.9188)
  line L175 (0.7784, 6.9188) -> (0.7784, 6.9285)
  spline S243 degree 2 poles (0.7784, 6.9285) (0.8092, 6.9707) (0.8659, 7.1133) (0.8659, 7.1838) knots 0 0 0 1 2 2 2
  spline S244 degree 2 poles (0.8659, 7.1838) (0.8659, 7.2251) (0.84, 7.3078) (0.81, 7.3353) knots 0 0 0 1 2 2 2
  spline S245 degree 2 poles (0.81, 7.3353) (0.78, 7.3621) (0.7087, 7.3904) (0.6544, 7.3904) knots 0 0 0 1 2 2 2
  spline S246 degree 2 poles (0.6544, 7.3904) (0.6001, 7.3904) (0.5296, 7.3588) (0.5094, 7.3305) knots 0 0 0 1 2 2 2
  spline S247 degree 2 poles (0.5094, 7.3305) (0.4891, 7.3021) (0.4737, 7.2251) (0.4737, 7.1797) knots 0 0 0 1 2 2 2
  line L176 (0.4737, 7.1797) -> (0.4737, 7.123)
  line L177 (0.4737, 7.123) -> (0.3627, 7.123)
  line L178 (0.3627, 7.123) -> (0.3627, 7.1676)
  spline S248 degree 2 poles (0.3627, 7.1676) (0.3627, 7.2575) (0.2768, 7.371) (0.1949, 7.371) knots 0 0 0 1 2 2 2
  spline S249 degree 2 poles (0.1949, 7.371) (0.1568, 7.371) (0.1026, 7.3418) (0.0863, 7.3183) knots 0 0 0 1 2 2 2
  spline S250 degree 2 poles (0.0863, 7.3183) (0.0693, 7.2932) (0.0556, 7.2316) (0.0556, 7.1968) knots 0 0 0 1 2 2 2
  spline S251 degree 2 poles (0.5766, 8.059) (0.7841, 8.059) (1.0985, 7.9261) (1.2371, 7.8086) knots 0 0 0 1 2 2 2
  line L179 (1.2371, 7.8086) -> (1.2371, 7.6546)
  line L180 (1.2371, 7.6546) -> (1.2306, 7.6546)
  spline S252 degree 2 poles (1.2306, 7.6546) (1.1844, 7.7065) (1.0491, 7.811) (0.968, 7.8499) knots 0 0 0 1 2 2 2
  spline S253 degree 2 poles (0.968, 7.8499) (0.8813, 7.8921) (0.6885, 7.9407) (0.5766, 7.9407) knots 0 0 0 1 2 2 2
  spline S254 degree 2 poles (0.5766, 7.9407) (0.4656, 7.9407) (0.2687, 7.8913) (0.1852, 7.8499) knots 0 0 0 1 2 2 2
  spline S255 degree 2 poles (0.1852, 7.8499) (0.1017, 7.8094) (-0.0312, 7.7057) (-0.0773, 7.6546) knots 0 0 0 1 2 2 2
  line L181 (-0.0773, 7.6546) -> (-0.0838, 7.6546)
  line L182 (-0.0838, 7.6546) -> (-0.0838, 7.8086)
  spline S256 degree 2 poles (-0.0838, 7.8086) (0.0547, 7.9253) (0.3675, 8.059) (0.5766, 8.059) knots 0 0 0 1 2 2 2
  point P0 (0, 0)
  dimension "d0" = 17.12
  dimension "d1" = 21.62
  constraints: 2 other
emboss "Emboss1" sketch "Sketch6" operation add depth 0.93 direction (0, -1, 0)
equation "\"d14\" = d13"
body "Solid1"
